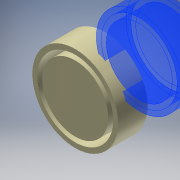
# Autodesk Inventor part: 실리콘틀_위
Saved by Autodesk Inventor 2017 (Build 210142000, 142)
## iProperties
Part Number: 실리콘틀_위
Material: 나일론, 이황화 몰리브덴
Document SubType Name: Modeling
Designer: minom
Density: 1.13 g/cm^3
Appearance: 나일론 6
Mass: 163.185 g
Surface Area: 313.986 cm^2
Volume: 144.411 cm^3
Author: minom
Autodesk Inventor part; units mm, degrees
ref_plane "YZ Plane" through (0, 0, 0) normal (1, 0, 0) x (0, 1, 0)
ref_plane "XZ Plane" through (0, 0, 0) normal (0, 1, 0) x (-1, 0, 0)
ref_plane "XY Plane" through (0, 0, 0) normal (0, 0, 1) x (1, 0, 0)
sketch "스케치1" plane through (0, 0, 0) normal (0, 1, 0) x (-1, 0, 0)
  circle A0 centre (0, 0) radius 43.5
  circle A1 centre (0, 0) radius 38.5
  circle A2 centre (0, 0) radius 33.5
  dimension "d0" = 87
  dimension "d1" = 77
  dimension "d2" = 67
  constraints: 3 centre point, 3 coincident
  measures "d0" diameter of A0
  measures "d1" diameter of A1
  measures "d2" diameter of A2
extrude "돌출1" add sketch "스케치1" along normal blind 30
